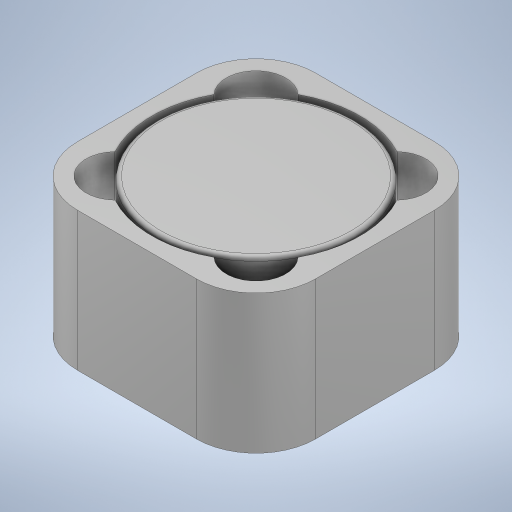
# Autodesk Inventor part: smd_power_inductor
Saved by Autodesk Inventor 2024.1 (Build 281209000, 209)
## iProperties
Created: 2025-02-20
Part Number: smd_power_inductor
Material: アルミニウム 6061
Document SubType Name: Modeling
Designer: hibik
Density: 2.7 g/cm^3
Appearance: アルミニウム - フラット
Author: hibik
Autodesk Inventor part; units mm, degrees
ref_plane "YZ Plane" through (0, 0, 0) normal (1, 0, 0) x (0, 1, 0)
ref_plane "XZ Plane" through (0, 0, 0) normal (0, 1, 0) x (-1, 0, 0)
ref_plane "XY Plane" through (0, 0, 0) normal (0, 0, 1) x (1, 0, 0)
sketch "スケッチ1" plane through (0, 0, 0) normal (0, 1, 0) x (-1, 0, 0)
  line L0 (-6, -6) -> (6, -6)
  line L1 (6, -6) -> (6, 6)
  line L2 (6, 6) -> (-6, 6)
  line L3 (-6, 6) -> (-6, -6)
  line L4 (-6, -6) -> (6, 6) construction
  line L5 (6, -6) -> (-6, 6) construction
  point P0 (0, 0)
  dimension "d0" = 12
  constraints: 12 end point, 2 midpoint, 2 parallel, 2 perpendicular, 1 horizontal
  measures "d0" distance of L0.end L1.end
extrude "押し出し1" add sketch "スケッチ1" along normal blind 7
fillet "フィレット1" radius 3 4 edges at (6, 3.5, 6) (6, 3.5, -6) (-6, 3.5, 6) (-6, 3.5, -6)
sketch "スケッチ2" plane through (0, 7, 0) normal (0, 1, 0) x (1, 0, 0)
  circle A0 centre (0, 0) radius 5
  circle A1 centre (-3.5355, 3.5355) radius 1.5
  circle A2 centre (3.5355, 3.5355) radius 1.5
  circle A3 centre (3.5355, -3.5355) radius 1.5
  circle A4 centre (-3.5355, -3.5355) radius 1.5
  line L0 (-3.5355, -3.5355) -> (3.5355, 3.5355) construction
  line L1 (-3.5355, 3.5355) -> (3.5355, -3.5355) construction
  line L2 (-8.4, 0) -> (8.4, 0) projected
  circle A5 centre (0, 0) radius 5.25
  point P0 (0, 0)
  point P1 (4.6181, -2.4972)
  point P2 (4.6181, 2.4972)
  point P3 (2.4972, 4.6181)
  point P4 (-2.4972, 4.6181)
  point P5 (-4.6181, 2.4972)
  point P6 (-4.6181, -2.4972)
  point P7 (-2.4972, -4.6181)
  point P8 (2.4972, -4.6181)
  dimension "d4" = 10
  dimension "d5" = 3
  dimension "d6" = 3
  dimension "d7" = 3
  dimension "d8" = 3
  dimension "d9" = 45
  dimension "d10" = 10.5
  constraints: 6 centre point, 4 end point, 4 midpoint, 4 point on circle, 2 coincident, 1 perpendicular
  measures "d4" diameter of A0
  measures "d5" diameter of A1
  measures "d6" diameter of A2
  measures "d7" diameter of A3
  measures "d8" diameter of A4
  measures "d9" angle of L2 L1
  measures "d10" diameter of A5
extrude "押し出し2" cut sketch "スケッチ2" against normal blind 3 contours L2 A5 A3 A0 | A0 A2 A5 L2 | A0 A2 A5 | A3 A5 A0 | L2 A5 A1 A0 | A0 A4 A5 L2 | A0 A1 A5 A2 | A5 A2 | A3 A5 A4 A0 | A3 A5 | A1 A5 A0 | A0 A4 A5 | A1 A5 | A5 A4
fillet "フィレット2" radius 0.2 1 edges at (-5, 7, 0)
